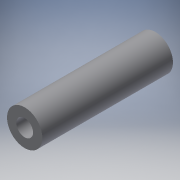
# Autodesk Inventor part: distanciador
Saved by Autodesk Inventor 2018 (Build 220112000, 112)
## iProperties
Created: 2018-03-07
Part Number: distanciador
Material: Generic
Document SubType Name: Modeling
Designer: isai
Density: 1 g/cm^3
Appearance: Default
Author: isai
Autodesk Inventor part; units mm, degrees
ref_plane "YZ Plane" through (0, 0, 0) normal (1, 0, 0) x (0, 1, 0)
sketch "Sketch1" plane through (0, 0, 0) normal (0, 0, 1) x (1, 0, 0)
  circle A0 centre (-8.4848, -18.3848) radius 1.8 projected
  circle A1 centre (-8.4848, -18.3848) radius 3.8
  point P0 (0, 0)
  dimension "d0" = 2
  dimension "d3" = 3.6
  constraints: 1 centre point
  measures "d0" radial gap between concentric circles of A0 A1
  measures "d3" diameter of A0
ref_plane "Work Plane1" through (-22.1, -32, 28.0512) normal (0, 0, -1) x (0, 1, 0)
ref_plane "Work Plane2" through (-39, -39, 10.6) normal (0, 0, -1) x (0, 1, 0)
extrude "Extrusion1" add sketch "Sketch1" along normal up to surface (10.6 mm away)
body "Solid1"
